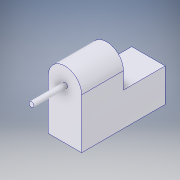
# Autodesk Inventor part: Motor
Saved by Autodesk Inventor 2018 (Build 220112000, 112)
## iProperties
Created: 2018-02-19
Part Number: Motor
Material: Generic
Document SubType Name: Modeling
Designer: Melda
Density: 1 g/cm^3
Appearance: Cool White
Author: Melda
Autodesk Inventor part; units mm, degrees
ref_plane "YZ Plane" through (0, 0, 0) normal (1, 0, 0) x (0, 1, 0)
ref_plane "XZ Plane" through (0, 0, 0) normal (0, 1, 0) x (-1, 0, 0)
ref_plane "XY Plane" through (0, 0, 0) normal (0, 0, 1) x (1, 0, 0)
sketch "Sketch1" plane through (0, 0, 0) normal (1, 0, 0) x (0, 1, 0)
  line L0 (14.6318, 23.7403) -> (-25.3682, 23.7403)
  line L1 (-25.3682, 23.7403) -> (-25.3682, -26.2597)
  line L2 (-25.3682, -26.2597) -> (-5.3682, -26.2597)
  line L3 (14.6318, -1.2597) -> (14.6318, 23.7403)
  line L4 (14.6318, -1.2597) -> (-5.3682, -1.2597)
  line L5 (-5.3682, -1.2597) -> (-5.3682, -26.2597)
  point P0 (0, 0)
  constraints: 12 end point, 2 horizontal, 2 parallel, 2 perpendicular
extrude "Extrusion1" add sketch "Sketch1" along normal blind 20
fillet "Fillet1" radius 10 2 edges at (20, 14.6318, 11.2403) (0, 14.6318, 11.2403)
sketch "Sketch3" plane through (0, -25.3682, 23.7403) normal (0, 0, 1) x (1, 0, 0)
  circle A0 centre (10, 30) radius 1.5
  arc A1 (20, 30) -> (0, 30) centre (10, 30) ccw projected
  point P0 (0, 25.3682)
  dimension "d5" = 3
  constraints: 1 centre point, 1 concentric
  measures "d5" diameter of A0
extrude "Extrusion2" add sketch "Sketch3" along normal blind 20
body "Solid1"
